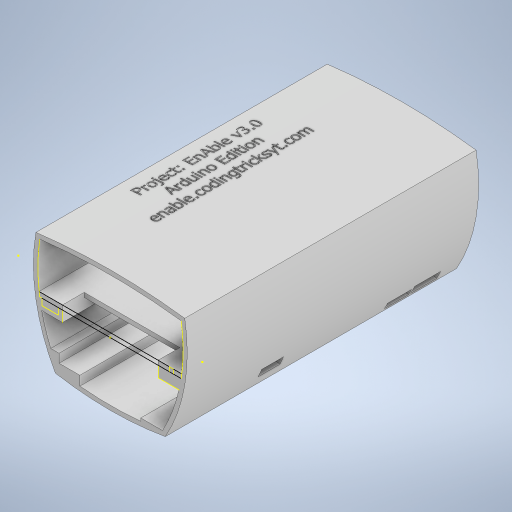
# Autodesk Inventor part: testingagain
Saved by Autodesk Inventor 2024 (Build 280153000, 153)
## iProperties
Created: 2022-11-19
Part Number: testingagain
Material: Generic
Document SubType Name: Modeling
Designer: jeron
Density: 1 g/cm^3
Appearance: Default
Author: jeron
Autodesk Inventor part; units mm, degrees
(part 1 of 2)
sketch "Sketch1" plane through (0, 0, 0) normal (0, 0, 1) x (1, 0, 0)
  line L0 (-32.5, 23) -> (32.5, 23)
  line L1 (32.5, 23) -> (32.5, 0)
  line L2 (-32.5, 0) -> (-32.5, 23)
  line L3 (-24, -18) -> (-24, 0)
  line L4 (24, -25) -> (24, -5)
  line L5 (0, -25) -> (24, -25)
  line L6 (0, -25) -> (-14, -25)
  line L7 (0, 23) -> (0, 25)
  line L8 (0, -25) -> (0, -27)
  arc A0 (-32.5, 23) -> (-24, -25) centre (42.3382, 11.5) ccw
  line L9 (-32.5, 0) -> (-31.5587, 0)
  line L10 (-24, 0) -> (-24, -5)
  line L11 (32.5, 0) -> (24, 0)
  line L12 (24, 0) -> (24, -5)
  line L13 (24, -5) -> (31.5587, -5)
  line L14 (24, -25) -> (15.6259, -25)
  line L15 (24, -25) -> (14, -25)
  line L16 (14, -25) -> (14, -26.3226)
  line L17 (-14, -25) -> (-14, -26.3226)
  arc A1 (32.5, 23) -> (-32.5, 23) centre (0, -240.0625) ccw
  arc A2 (24, -25) -> (32.5, 23) centre (-42.3382, 11.5) ccw
  arc A3 (-24, -25) -> (24, -25) centre (0, 118) ccw
  arc A4 (-34.2324, 24.7969) -> (-25.28, -26.8099) centre (42.3382, 11.5) ccw
  arc A5 (-25.28, -26.8099) -> (25.28, -26.8099) centre (0, 118) ccw
  arc A6 (25.28, -26.8099) -> (34.2324, 24.7969) centre (-42.3382, 11.5) ccw
  arc A7 (34.2324, 24.7969) -> (-34.2324, 24.7969) centre (0, -240.0625) ccw
  line L18 (-14, -25) -> (-14, -22)
  line L19 (-14, -22) -> (-25.5644, -22)
  line L20 (-24, -5) -> (-22, -5)
  line L21 (-22, -5) -> (-22, 0)
  line L22 (-31.5587, -5) -> (-31.5587, 0)
  line L23 (-32.5, 0) -> (-31.5587, 0)
  line L24 (-24, 0) -> (32.5, 0)
  line L25 (24, -5) -> (22, -5)
  line L26 (22, -5) -> (22, 0)
  line L27 (24, 0) -> (27, 0)
  line L28 (27, 0) -> (27, 2)
  line L29 (27, 2) -> (29, 2)
  line L30 (29, 2) -> (29, 0)
  line L31 (27, 0) -> (29, 0)
  line L32 (-25.5644, -22) -> (-23.5644, -22)
  line L33 (-23.5644, -22) -> (-23.5644, -18)
  line L34 (-23.5644, -18) -> (-27.3953, -18)
  line L35 (-24, -5) -> (-24, -3)
  line L36 (-24, -3) -> (-31.977, -3)
  line L37 (-24, -5) -> (-31.5587, -5)
  line L38 (0, 0) -> (0, -1.7837)
  point P0 (0, -28)
  point P1 (0, 26)
  point P2 (27, 0)
  point P3 (29, 0)
  point P4 (-31.5587, -3)
  point P5 (0, -29)
  point P6 (0, -27)
  point P7 (0, 27)
  point P8 (0, 25)
  dimension "d19" = 65
  dimension "d20" = 23
  dimension "d30" = 65
  dimension "d39" = 48
  dimension "d40" = 25
  dimension "d41" = 8.5
  dimension "d42" = 8.5
  dimension "d43" = 2
  dimension "d44" = 2
  dimension "d45" = 54
  dimension "d46" = 5
  dimension "d47" = 5
  dimension "d48" = 10
  dimension "d49" = 10
  dimension "d54" = 3
  dimension "d55" = 2
  dimension "d56" = 2
  dimension "d68" = 3
  dimension "d69" = 2
  dimension "d70" = 2
  dimension "d84" = 2
  dimension "d85" = 4
  dimension "d88" = 2
  dimension "d123" = 23
  dimension "d124" = 25
  dimension "d125" = 32.5
  dimension "d126" = 2
  dimension "d127" = 2
  constraints: 78 end point, 28 point on circle, 14 perpendicular, 12 point on line, 8 centre point, 7 horizontal, 4 collinear, 4 vertical, 1 midpoint, 1 parallel, 3 other
  measures "d19" distance of L0.start L0.end
  measures "d20" distance of L0.end L1.end
  measures "d30" distance of L1.end L2.start
  measures "d39" distance of L11.end L3.end
  measures "d40" distance of L4.start L11.end
  measures "d41" distance of L11.end L1.end
  measures "d42" distance of L2.start L3.end
  measures "d43" distance of L7.start L7.end
  measures "d44" distance of L5.start L8.end
  measures "d45" distance of point (0, -28) point (0, 26)
  measures "d46" distance of L3.end L10.end
  measures "d47" distance of L4.end L11.end
  measures "d48" distance of L14.start L15.end
  measures "d49" distance of L6.end A0.end
  measures "d54" distance of L6.end L18.end
  measures "d55" distance of L10.end L20.end
  measures "d56" distance of L4.end L25.end
  measures "d68" distance of L11.end L27.end
  measures "d69" distance of L27.end L28.end
  measures "d70" distance of L28.end L29.end
  measures "d84" distance of L19.end L32.end
  measures "d85" distance of L32.end L33.end
  measures "d88" distance of L10.end L35.end
  measures "d123" distance between parallel lines of L0 L24
  measures "d124" distance between parallel lines of L6 L24
  measures "d125" distance of L38.start L1.end
  measures "d126" distance of point (0, -29) point (0, -27)
  measures "d127" distance of point (0, 27) point (0, 25)
extrude "Extrusion3" add sketch "Sketch1" along normal blind 100 contours L9 L22 L36 A0 | L36 L22 A0 | A2 L13 L12 L11 | L3 L24 L21 L20 | L25 L26 L24 L12 | A3 L16 L5 | L19 L18 L17 A3 A0 | A7 A6 A5 A4
extrude "Extrusion4" add sketch "Sketch1" against normal blind 2 contours A1 L7 L0 | L0 L1 L11 L30 L29 L28 L24 L3 L36 L22 L9 L2 | L2 A0 | L7 A1 L0 | L9 L22 L36 A0 | A2 L1 | L36 L22 A0 | A2 L13 L12 L11 | L37 L3 L34 A0 | L22 L36 L3 L37 | L11 L28 L29 L30 | A2 L4 L13 | L34 L33 L19 A0 | L20 L21 L24 L26 L25 L4 L5 L6 L18 L19 L33 L34 L3 | L3 L24 L21 L20 | L25 L26 L24 L12 | A3 L16 L5 | L19 L18 L17 A3 A0 | A3 L8 L5 L16 | A3 L17 L6 L8 | A7 A6 A5 A4
ref_plane "Work Plane2" through (0, 27, 100) normal (0, 1, 0) x (-1, 0, 0)
sketch "Sketch3" plane through (0, 0, 0) normal (0, 0, 1) x (1, 0, 0)
  point P0 (0, 0)
ref_plane "Work Plane4" through (34.2348, -1.7834, -2) normal (0.9852847, -0.1709212, 0) x (0.1709212, 0.9852847, 0)
sketch "Sketch5" plane through (34.2348, -1.7834, -2) normal (0.9852847, -0.1709212, 0) x (0.1709212, 0.9852847, 0)
  line L0 (-24.6243, 2) -> (-24.6243, 102) projected
  line L1 (-24.6243, 2) -> (-24.6243, 10)
  line L2 (-24.6243, 10) -> (-20.6243, 10)
  line L3 (-20.6243, 10) -> (-20.6243, 22)
  line L4 (-20.6243, 22) -> (-24.6243, 22)
  line L5 (-24.6243, 22) -> (-24.6243, 23)
  line L6 (-24.6243, 23) -> (-21.6243, 23)
  line L7 (-21.6243, 23) -> (-21.6243, 34)
  line L8 (-21.6243, 34) -> (-24.6243, 34)
  line L9 (-24.6243, 2) -> (-24.6243, 84)
  line L10 (-24.6243, 84) -> (-16.6243, 84)
  line L11 (-16.6243, 84) -> (-16.6243, 94)
  line L12 (-16.6243, 94) -> (-24.6243, 94)
  line L13 (-24.6243, 84) -> (-20.6243, 84)
  line L14 (-20.6243, 84) -> (-20.6243, 94)
  point P0 (-4.0943, 2)
  dimension "d76" = 8
  dimension "d77" = 4
  dimension "d78" = 12
  dimension "d79" = 1
  dimension "d80" = 3
  dimension "d81" = 11
  dimension "d91" = 82
  dimension "d92" = 8
  dimension "d93" = 10
  dimension "d94" = 4
  constraints: 28 end point, 8 perpendicular, 6 point on line, 2 midpoint, 1 vertical
  measures "d76" distance of L0.start L1.end
  measures "d77" distance of L1.end L2.end
  measures "d78" distance of L2.end L3.end
  measures "d79" distance of L4.end L5.end
  measures "d80" distance of L5.end L6.end
  measures "d81" distance of L6.end L7.end
  measures "d91" distance of L0.start L9.end
  measures "d92" distance of L9.end L10.end
  measures "d93" distance of L10.end L11.end
  measures "d94" distance of L9.end L13.end
extrude "Extrusion7" cut sketch "Sketch5" against normal blind 10 contours L0 L4 L3 L2 | L0 L8 L7 L6 | L14 L12 L11 L10
extrude "Extrusion8" add sketch "Sketch1" along normal up to surface (100 mm away) contours L11 L28 L29 L30 | L34 L33 L19 A0
extrude "Extrusion9" add sketch "Sketch1" along normal up to surface (100 mm away) contours L22 L36 L3 L37
ref_plane "Work Plane5" through (-34.2348, -1.7834, 100) normal (-0.9852847, -0.1709212, 0) x (0.1709212, -0.9852847, 0)
sketch "Sketch6" plane through (-34.2348, -1.7834, 100) normal (-0.9852847, -0.1709212, 0) x (0.1709212, -0.9852847, 0)
  line L0 (17.147, 0) -> (17.147, -100) projected
  line L1 (17.147, -100) -> (17.147, -18)
  line L2 (17.147, -18) -> (13.147, -18)
  line L3 (13.147, -18) -> (13.147, -8)
  line L4 (13.147, -8) -> (17.147, -8)
  point P0 (4.0943, -100)
  dimension "d95" = 82
  dimension "d96" = 4
  dimension "d97" = 10
  constraints: 8 end point, 3 perpendicular, 2 point on line
  measures "d95" distance of L0.end L1.end
  measures "d96" distance of L1.end L2.end
  measures "d97" distance of L2.end L3.end
extrude "Extrusion10" cut sketch "Sketch6" against normal blind 10
ref_plane "Work Plane6" through (34.2324, 24.7969, 100) normal (0, 0, 1) x (1, 0, 0)
sketch "Sketch7" plane through (34.2324, 24.7969, 100) normal (0, 0, 1) x (1, 0, 0)
  arc A0 (0, 0) -> (-68.4649, 0) centre (-34.2324, -264.8594) ccw projected
  arc A1 (-68.4649, 0) -> (-59.5124, -51.6069) centre (8.1058, -13.2969) ccw projected
  arc A2 (-66.7324, -1.7969) -> (-66.7324, -24.7969) centre (8.1058, -13.2969) ccw projected
  arc A3 (-1.7324, -1.7969) -> (-66.7324, -1.7969) centre (-34.2324, -264.8594) ccw projected
  arc A4 (-8.9524, -51.6069) -> (0, 0) centre (-76.5707, -13.2969) ccw projected
  arc A5 (-1.7324, -24.7969) -> (-1.7324, -1.7969) centre (-76.5707, -13.2969) ccw projected
  line L0 (-1.7324, -24.7969) -> (-5.2324, -24.7969) projected
  line L1 (-5.2324, -22.7969) -> (-5.2324, -24.7969) projected
  line L2 (-7.2324, -22.7969) -> (-5.2324, -22.7969) projected
  line L3 (-7.2324, -24.7969) -> (-7.2324, -22.7969) projected
  line L4 (-7.2324, -24.7969) -> (-12.2324, -24.7969) projected
  line L5 (-12.2324, -24.7969) -> (-12.2324, -29.7969) projected
  line L6 (-12.2324, -29.7969) -> (-2.6737, -29.7969) projected
  arc A6 (-10.2324, -49.7969) -> (-2.6737, -29.7969) centre (-76.5707, -13.2969) ccw projected
  line L7 (-65.7912, -24.7969) -> (-66.7324, -24.7969) projected
  line L8 (-65.7912, -27.7969) -> (-65.7912, -24.7969) projected
  line L9 (-65.7912, -27.7969) -> (-58.2324, -27.7969) projected
  line L10 (-58.2324, -24.7969) -> (-58.2324, -27.7969) projected
  line L11 (-56.2324, -24.7969) -> (-58.2324, -24.7969) projected
  line L12 (-56.2324, -29.7969) -> (-56.2324, -24.7969) projected
  line L13 (-56.2324, -29.7969) -> (-65.7912, -29.7969) projected
  arc A7 (-65.7912, -29.7969) -> (-61.6277, -42.7969) centre (8.1058, -13.2969) ccw projected
  line L14 (-61.6277, -42.7969) -> (-57.7968, -42.7969) projected
  line L15 (-57.7968, -42.7969) -> (-57.7968, -46.7969) projected
  line L16 (-48.2324, -46.7969) -> (-57.7968, -46.7969) projected
  line L17 (-48.2324, -51.1195) -> (-48.2324, -46.7969) projected
  arc A8 (-48.2324, -51.1195) -> (-20.2324, -51.1195) centre (-34.2324, 93.2031) ccw projected
  line L18 (-20.2324, -49.7969) -> (-20.2324, -51.1195) projected
  line L19 (-10.2324, -49.7969) -> (-20.2324, -49.7969) projected
  arc A9 (-59.5124, -51.6069) -> (-8.9524, -51.6069) centre (-34.2324, 93.2031) ccw projected
  point P0 (-34.2324, -24.7969)
extrude "Extrusion11" add sketch "Sketch7" along normal blind 32
sketch "Sketch8" plane through (0, 0, -2) normal (0, 0, -1) x (-1, 0, 0)
  circle A0 centre (0, 0) radius 16
  arc A1 (30.7676, 23.2082) -> (-24.2324, 23.89) centre (0, -240.0625) ccw projected
  line L0 (30.7676, 23.2082) -> (7.9501, 23.2082)
  line L1 (7.9501, 23.2082) -> (7.9501, 13.8851)
  line L2 (15.0321, 5.4805) -> (30.7676, 5.4805)
  line L3 (30.7676, 5.4805) -> (30.7676, 23.2082)
  circle A2 centre (0, 10) radius 1.5
  circle A3 centre (0, -10) radius 1.5
  dimension "d102" = 32
  dimension "d104" = 3
  dimension "d106" = 3
  dimension "d121" = 10
  dimension "d122" = 10
  dimension "d128" = 7.9501
  dimension "d129" = 13.8851
  dimension "d130" = 22.8175
  dimension "d131" = 17.7278
  constraints: 8 end point, 3 centre point, 2 horizontal, 2 perpendicular, 2 point on circle, 1 coincident
  measures "d102" diameter of A0
  measures "d104" diameter of A2
  measures "d106" diameter of A3
  measures "d121" distance of point (0, 0) A2.centre
  measures "d122" distance of point (0, 0) A3.centre
  measures "d128" horizontal distance of point (0, 0) L1.end
  measures "d129" vertical distance of point (0, 0) L1.end
  measures "d130" distance of L0.end L0.start
  measures "d131" distance of L2.end L0.start
extrude "Extrusion12" cut sketch "Sketch8" against normal up to surface (2 mm away) contours A0 L1 L0 L3 L2 | A2 | A3
sketch "Sketch9" plane through (34.2324, 24.7969, 132) normal (0, 0, 1) x (1, 0, 0)
  point P0 (-34.2324, -24.7969)
sketch "Sketch11" plane through (34.2324, 24.7969, 132) normal (0, 0, 1) x (1, 0, 0)
  line L0 (-65.7912, -24.7969) -> (-66.7324, -24.7969) projected
  line L1 (-7.2324, -24.7969) -> (-12.2324, -24.7969) projected
  line L2 (-65.7912, -24.7969) -> (-7.2324, -24.7969)
  arc A0 (-1.7324, -24.7969) -> (-1.7324, -1.7969) centre (-76.5707, -13.2969) ccw projected
  line L3 (-7.2324, -24.7969) -> (-1.7324, -24.7969)
  line L4 (-56.2324, -29.7969) -> (-56.2324, -24.7969) projected
  line L5 (-12.2324, -29.7969) -> (-2.6737, -29.7969) projected
  line L6 (-58.2324, -27.7969) -> (-65.7912, -27.7969) projected
  line L7 (-58.2324, -24.7969) -> (-58.2324, -27.7969) projected
  line L8 (-65.7912, -27.7969) -> (-65.7912, -24.7969) projected
  line L9 (-7.2324, -22.7969) -> (-7.2324, -24.7969) projected
  line L10 (-5.2324, -22.7969) -> (-7.2324, -22.7969) projected
  line L11 (-5.2324, -24.7969) -> (-5.2324, -22.7969) projected
  line L12 (-12.2324, -24.7969) -> (-12.2324, -29.7969) projected
  line L13 (-5.2324, -22.7969) -> (-1.4524, -22.7969)
  line L14 (-7.2324, -22.7969) -> (-67.0125, -22.7969)
  arc A1 (-66.7324, -1.7969) -> (-66.7324, -24.7969) centre (8.1058, -13.2969) ccw projected
  point P0 (-34.2324, -24.7969)
  constraints: 8 end point, 2 point on circle, 1 collinear, 1 horizontal, 1 parallel, 1 point on line
extrude "Extrusion15" add sketch "Sketch11" against normal up to surface (132 mm away) contours L2 L7 L6 L8
ref_plane "Work Plane7" through (0, 27, -2) normal (0, 1, 0) x (-1, 0, 0)
sketch "Sketch14" plane through (0, 27, -2) normal (0, 1, 0) x (-1, 0, 0)
  line L0 (28.7956, 103.5089) -> (28.7956, 32.4114) construction
  line L1 (28.7956, 32.4114) -> (-135.0036, 32.4114) construction
  line L2 (-135.0036, 32.4114) -> (-135.0036, 103.5089) construction
  line L3 (-135.0036, 103.5089) -> (28.7956, 103.5089) construction
  spline S0 degree 2 poles (27.1788, 93.3054) (26.8759, 93.3054) (26.3306, 93.5212) (26.1413, 93.7143) knots 0 0 0 1 2 2 2
  spline S1 degree 2 poles (26.1413, 93.7143) (25.9027, 93.9566) (25.6566, 94.6117) (25.6566, 95.1115) knots 0 0 0 1 2 2 2
  line L4 (25.6566, 95.1115) -> (25.6566, 95.6379)
  line L5 (25.6566, 95.6379) -> (23.9148, 95.6379)
  line L6 (23.9148, 95.6379) -> (23.9148, 96.2588)
  line L7 (23.9148, 96.2588) -> (28.5874, 96.2588)
  line L8 (28.5874, 96.2588) -> (28.5874, 95.085)
  spline S2 degree 2 poles (28.5874, 95.085) (28.5874, 94.6685) (28.4511, 94.0854) (28.2958, 93.862) knots 0 0 0 1 2 2 2
  spline S3 degree 2 poles (28.2958, 93.862) (28.1178, 93.6007) (27.5688, 93.3054) (27.1788, 93.3054) knots 0 0 0 1 2 2 2
  spline S4 degree 2 poles (27.1598, 93.9528) (27.4022, 93.9528) (27.7581, 94.1195) (27.8717, 94.2898) knots 0 0 0 1 2 2 2
  spline S5 degree 2 poles (27.8717, 94.2898) (27.9702, 94.4375) (28.0497, 94.8313) (28.0497, 95.1229) knots 0 0 0 1 2 2 2
  line L9 (28.0497, 95.1229) -> (28.0497, 95.6379)
  line L10 (28.0497, 95.6379) -> (26.1867, 95.6379)
  line L11 (26.1867, 95.6379) -> (26.1867, 95.2138)
  spline S6 degree 2 poles (26.1867, 95.2138) (26.1867, 94.8351) (26.3079, 94.3694) (26.4669, 94.2179) knots 0 0 0 1 2 2 2
  spline S7 degree 2 poles (26.4669, 94.2179) (26.607, 94.0778) (26.9364, 93.9528) (27.1598, 93.9528) knots 0 0 0 1 2 2 2
  line L12 (26.7888, 90.9009) -> (26.7888, 90.9312)
  spline S8 degree 2 poles (26.7888, 90.9312) (26.8077, 90.9994) (26.8153, 91.147) (26.8153, 91.2493) knots 0 0 0 1 2 2 2
  spline S9 degree 2 poles (26.8153, 91.2493) (26.8153, 91.4878) (26.607, 91.9573) (26.4025, 92.1694) knots 0 0 0 1 2 2 2
  line L13 (26.4025, 92.1694) -> (23.9148, 92.1694)
  line L14 (23.9148, 92.1694) -> (23.9148, 92.7601)
  line L15 (23.9148, 92.7601) -> (27.4211, 92.7601)
  line L16 (27.4211, 92.7601) -> (27.4211, 92.1694)
  line L17 (27.4211, 92.1694) -> (26.8986, 92.1694)
  spline S10 degree 2 poles (26.8986, 92.1694) (27.1863, 91.8475) (27.4211, 91.3666) (27.4211, 91.1395) knots 0 0 0 1 2 2 2
  spline S11 degree 2 poles (27.4211, 91.1395) (27.4211, 91.0486) (27.4135, 90.9577) (27.4022, 90.9009) knots 0 0 0 1 2 2 2
  line L18 (27.4022, 90.9009) -> (26.7888, 90.9009)
  spline S12 degree 2 poles (25.6679, 87.5612) (24.7819, 87.5612) (23.8163, 88.4131) (23.8163, 89.125) knots 0 0 0 1 2 2 2
  spline S13 degree 2 poles (23.8163, 89.125) (23.8163, 89.8558) (24.8122, 90.6926) (25.6679, 90.6926) knots 0 0 0 1 2 2 2
  spline S14 degree 2 poles (25.6679, 90.6926) (26.5464, 90.6926) (27.5196, 89.8293) (27.5196, 89.125) knots 0 0 0 1 2 2 2
  spline S15 degree 2 poles (27.5196, 89.125) (27.5196, 88.4131) (26.5502, 87.5612) (25.6679, 87.5612) knots 0 0 0 1 2 2 2
  spline S16 degree 2 poles (25.6679, 88.1708) (26.3495, 88.1708) (27.0122, 88.6668) (27.0122, 89.125) knots 0 0 0 1 2 2 2
  spline S17 degree 2 poles (27.0122, 89.125) (27.0122, 89.5832) (26.3495, 90.083) (25.6679, 90.083) knots 0 0 0 1 2 2 2
  spline S18 degree 2 poles (25.6679, 90.083) (25.0053, 90.083) (24.3237, 89.5832) (24.3237, 89.125) knots 0 0 0 1 2 2 2
  spline S19 degree 2 poles (24.3237, 89.125) (24.3237, 88.6706) (24.9939, 88.1708) (25.6679, 88.1708) knots 0 0 0 1 2 2 2
  spline S20 degree 2 poles (23.8163, 86.0011) (23.2181, 86.0011) (22.5895, 86.6448) (22.5895, 87.209) knots 0 0 0 1 2 2 2
  spline S21 degree 2 poles (22.5895, 87.209) (22.5895, 87.3075) (22.6084, 87.5498) (22.6274, 87.6672) knots 0 0 0 1 2 2 2
  line L19 (22.6274, 87.6672) -> (23.1575, 87.6672)
  line L20 (23.1575, 87.6672) -> (23.1575, 87.6331)
  spline S22 degree 2 poles (23.1575, 87.6331) (23.1423, 87.565) (23.112, 87.3984) (23.112, 87.3226) knots 0 0 0 1 2 2 2
  spline S23 degree 2 poles (23.112, 87.3226) (23.112, 87.0879) (23.2294, 86.7812) (23.3544, 86.7092) knots 0 0 0 1 2 2 2
  spline S24 degree 2 poles (23.3544, 86.7092) (23.468, 86.6373) (23.8125, 86.5918) (24.0587, 86.5918) knots 0 0 0 1 2 2 2
  line L21 (24.0587, 86.5918) -> (26.9327, 86.5918)
  line L22 (26.9327, 86.5918) -> (26.9327, 87.2242)
  line L23 (26.9327, 87.2242) -> (27.4211, 87.2242)
  line L24 (27.4211, 87.2242) -> (27.4211, 86.0011)
  line L25 (27.4211, 86.0011) -> (23.8163, 86.0011)
  line L26 (28.0042, 85.9973) -> (28.0042, 86.6676)
  line L27 (28.0042, 86.6676) -> (28.6177, 86.6676)
  line L28 (28.6177, 86.6676) -> (28.6177, 85.9973)
  line L29 (28.6177, 85.9973) -> (28.0042, 85.9973)
  spline S25 degree 2 poles (23.8353, 83.6232) (23.8353, 84.4638) (24.7781, 85.3877) (25.649, 85.3877) knots 0 0 0 1 2 2 2
  spline S26 degree 2 poles (25.649, 85.3877) (26.5048, 85.3877) (27.5196, 84.4903) (27.5196, 83.7671) knots 0 0 0 1 2 2 2
  spline S27 degree 2 poles (27.5196, 83.7671) (27.5196, 83.4414) (27.3302, 82.9378) (27.1296, 82.7523) knots 0 0 0 1 2 2 2
  spline S28 degree 2 poles (27.1296, 82.7523) (26.9289, 82.563) (26.3495, 82.3623) (25.9292, 82.3623) knots 0 0 0 1 2 2 2
  line L30 (25.9292, 82.3623) -> (25.6074, 82.3623)
  line L31 (25.6074, 82.3623) -> (25.6074, 84.7894)
  spline S29 degree 2 poles (25.6074, 84.7894) (24.9977, 84.7894) (24.3502, 84.176) (24.3502, 83.6308) knots 0 0 0 1 2 2 2
  spline S30 degree 2 poles (24.3502, 83.6308) (24.3502, 83.4376) (24.4373, 83.0628) (24.5055, 82.9113) knots 0 0 0 1 2 2 2
  spline S31 degree 2 poles (24.5055, 82.9113) (24.5812, 82.7523) (24.7137, 82.5327) (24.7743, 82.4607) knots 0 0 0 1 2 2 2
  line L32 (24.7743, 82.4607) -> (24.7743, 82.4266)
  line L33 (24.7743, 82.4266) -> (24.1306, 82.4266)
  spline S32 degree 2 poles (24.1306, 82.4266) (24.089, 82.5289) (23.9678, 82.8394) (23.9337, 82.9605) knots 0 0 0 1 2 2 2
  spline S33 degree 2 poles (23.9337, 82.9605) (23.8845, 83.1309) (23.8353, 83.4111) (23.8353, 83.6232) knots 0 0 0 1 2 2 2
  spline S34 degree 2 poles (26.058, 82.9378) (26.2965, 82.9454) (26.6449, 83.0438) (26.7623, 83.1385) knots 0 0 0 1 2 2 2
  spline S35 degree 2 poles (26.7623, 83.1385) (26.8948, 83.2407) (27.0349, 83.5626) (27.0349, 83.8011) knots 0 0 0 1 2 2 2
  spline S36 degree 2 poles (27.0349, 83.8011) (27.0349, 84.0359) (26.8948, 84.3653) (26.7585, 84.5017) knots 0 0 0 1 2 2 2
  spline S37 degree 2 poles (26.7585, 84.5017) (26.6184, 84.6342) (26.2814, 84.7705) (26.058, 84.7894) knots 0 0 0 1 2 2 2
  line L34 (26.058, 84.7894) -> (26.058, 82.9378)
  spline S38 degree 2 poles (23.8353, 80.3705) (23.8353, 80.7341) (24.0587, 81.3361) (24.2859, 81.5519) knots 0 0 0 1 2 2 2
  spline S39 degree 2 poles (24.2859, 81.5519) (24.5093, 81.7678) (25.1984, 82.0063) (25.6604, 82.0063) knots 0 0 0 1 2 2 2
  spline S40 degree 2 poles (25.6604, 82.0063) (26.1223, 82.0063) (26.7963, 81.7602) (27.0235, 81.5519) knots 0 0 0 1 2 2 2
  spline S41 degree 2 poles (27.0235, 81.5519) (27.2545, 81.3437) (27.5006, 80.7265) (27.5006, 80.3705) knots 0 0 0 1 2 2 2
  spline S42 degree 2 poles (27.5006, 80.3705) (27.5006, 80.0828) (27.3378, 79.5451) (27.2318, 79.3368) knots 0 0 0 1 2 2 2
  line L35 (27.2318, 79.3368) -> (26.5691, 79.3368)
  line L36 (26.5691, 79.3368) -> (26.5691, 79.3709)
  spline S43 degree 2 poles (26.5691, 79.3709) (26.6222, 79.4353) (26.7585, 79.6322) (26.8304, 79.7723) knots 0 0 0 1 2 2 2
  spline S44 degree 2 poles (26.8304, 79.7723) (26.891, 79.8972) (26.9857, 80.2304) (26.9857, 80.3819) knots 0 0 0 1 2 2 2
  spline S45 degree 2 poles (26.9857, 80.3819) (26.9857, 80.8401) (26.2927, 81.3967) (25.6604, 81.3967) knots 0 0 0 1 2 2 2
  spline S46 degree 2 poles (25.6604, 81.3967) (25.0432, 81.3967) (24.3502, 80.859) (24.3502, 80.3819) knots 0 0 0 1 2 2 2
  spline S47 degree 2 poles (24.3502, 80.3819) (24.3502, 80.0941) (24.5888, 79.5716) (24.7743, 79.3709) knots 0 0 0 1 2 2 2
  line L37 (24.7743, 79.3709) -> (24.7743, 79.3368)
  line L38 (24.7743, 79.3368) -> (24.1117, 79.3368)
  spline S48 degree 2 poles (24.1117, 79.3368) (24.07, 79.4239) (23.9526, 79.689) (23.9261, 79.795) knots 0 0 0 1 2 2 2
  spline S49 degree 2 poles (23.9261, 79.795) (23.8807, 79.9465) (23.8353, 80.185) (23.8353, 80.3705) knots 0 0 0 1 2 2 2
  spline S50 degree 2 poles (23.8466, 77.7389) (23.8466, 78.2198) (24.3957, 78.7613) (24.9902, 78.7613) knots 0 0 0 1 2 2 2
  line L39 (24.9902, 78.7613) -> (26.9327, 78.7613)
  line L40 (26.9327, 78.7613) -> (26.9327, 79.1589)
  line L41 (26.9327, 79.1589) -> (27.4211, 79.1589)
  line L42 (27.4211, 79.1589) -> (27.4211, 78.7613)
  line L43 (27.4211, 78.7613) -> (28.4283, 78.7613)
  line L44 (28.4283, 78.7613) -> (28.4283, 78.1706)
  line L45 (28.4283, 78.1706) -> (27.4211, 78.1706)
  line L46 (27.4211, 78.1706) -> (27.4211, 77.0838)
  line L47 (27.4211, 77.0838) -> (26.9327, 77.0838)
  line L48 (26.9327, 77.0838) -> (26.9327, 78.1706)
  line L49 (26.9327, 78.1706) -> (25.2628, 78.1706)
  spline S51 degree 2 poles (25.2628, 78.1706) (24.9977, 78.1706) (24.7062, 78.1516) (24.5812, 78.0873) knots 0 0 0 1 2 2 2
  spline S52 degree 2 poles (24.5812, 78.0873) (24.4714, 78.0343) (24.3616, 77.7957) (24.3616, 77.5912) knots 0 0 0 1 2 2 2
  spline S53 degree 2 poles (24.3616, 77.5912) (24.3616, 77.4473) (24.4487, 77.1785) (24.4752, 77.1179) knots 0 0 0 1 2 2 2
  line L50 (24.4752, 77.1179) -> (24.4752, 77.0838)
  line L51 (24.4752, 77.0838) -> (23.9451, 77.0838)
  spline S54 degree 2 poles (23.9451, 77.0838) (23.8996, 77.2504) (23.8466, 77.5912) (23.8466, 77.7389) knots 0 0 0 1 2 2 2
  line L52 (23.9148, 75.5654) -> (23.9148, 76.3152)
  line L53 (23.9148, 76.3152) -> (24.8084, 76.3152)
  line L54 (24.8084, 76.3152) -> (24.8084, 75.5654)
  line L55 (24.8084, 75.5654) -> (23.9148, 75.5654)
  line L56 (26.5275, 75.5654) -> (26.5275, 76.3152)
  line L57 (26.5275, 76.3152) -> (27.4211, 76.3152)
  line L58 (27.4211, 76.3152) -> (27.4211, 75.5654)
  line L59 (27.4211, 75.5654) -> (26.5275, 75.5654)
  line L60 (23.9148, 72.3242) -> (28.5874, 72.3242)
  line L61 (28.5874, 72.3242) -> (28.5874, 69.401)
  line L62 (28.5874, 69.401) -> (28.0345, 69.401)
  line L63 (28.0345, 69.401) -> (28.0345, 71.7032)
  line L64 (28.0345, 71.7032) -> (26.7547, 71.7032)
  line L65 (26.7547, 71.7032) -> (26.7547, 69.5562)
  line L66 (26.7547, 69.5562) -> (26.2019, 69.5562)
  line L67 (26.2019, 69.5562) -> (26.2019, 71.7032)
  line L68 (26.2019, 71.7032) -> (24.4676, 71.7032)
  line L69 (24.4676, 71.7032) -> (24.4676, 69.401)
  line L70 (24.4676, 69.401) -> (23.9148, 69.401)
  line L71 (23.9148, 69.401) -> (23.9148, 72.3242)
  line L72 (23.9148, 66.012) -> (23.9148, 66.6027)
  line L73 (23.9148, 66.6027) -> (25.9141, 66.6027)
  spline S55 degree 2 poles (25.9141, 66.6027) (26.1564, 66.6027) (26.5729, 66.6481) (26.6979, 66.7163) knots 0 0 0 1 2 2 2
  spline S56 degree 2 poles (26.6979, 66.7163) (26.8304, 66.7882) (26.9592, 67.0457) (26.9592, 67.2654) knots 0 0 0 1 2 2 2
  spline S57 degree 2 poles (26.9592, 67.2654) (26.9592, 67.485) (26.7244, 67.9507) (26.5351, 68.1741) knots 0 0 0 1 2 2 2
  line L74 (26.5351, 68.1741) -> (23.9148, 68.1741)
  line L75 (23.9148, 68.1741) -> (23.9148, 68.7648)
  line L76 (23.9148, 68.7648) -> (27.4211, 68.7648)
  line L77 (27.4211, 68.7648) -> (27.4211, 68.1741)
  line L78 (27.4211, 68.1741) -> (27.0311, 68.1741)
  spline S58 degree 2 poles (27.0311, 68.1741) (27.2697, 67.9091) (27.5196, 67.3979) (27.5196, 67.1101) knots 0 0 0 1 2 2 2
  spline S59 degree 2 poles (27.5196, 67.1101) (27.5196, 66.5951) (26.838, 66.012) (26.1905, 66.012) knots 0 0 0 1 2 2 2
  line L79 (26.1905, 66.012) -> (23.9148, 66.012)
  line L80 (23.9148, 65.6409) -> (28.5874, 64.0657)
  line L81 (28.5874, 64.0657) -> (28.5874, 63.3008)
  line L82 (28.5874, 63.3008) -> (23.9148, 61.7257)
  line L83 (23.9148, 61.7257) -> (23.9148, 62.3807)
  line L84 (23.9148, 62.3807) -> (25.2211, 62.8048)
  line L85 (25.2211, 62.8048) -> (25.2211, 64.5883)
  line L86 (25.2211, 64.5883) -> (23.9148, 65.0124)
  line L87 (23.9148, 65.0124) -> (23.9148, 65.6409)
  line L88 (25.7513, 62.9752) -> (27.9512, 63.6984)
  line L89 (27.9512, 63.6984) -> (25.7513, 64.4179)
  line L90 (25.7513, 64.4179) -> (25.7513, 62.9752)
  spline S60 degree 2 poles (25.7247, 58.3897) (24.8652, 58.3897) (23.8163, 59.2228) (23.8163, 59.8513) knots 0 0 0 1 2 2 2
  spline S61 degree 2 poles (23.8163, 59.8513) (23.8163, 60.1353) (23.9564, 60.5405) (24.0776, 60.7374) knots 0 0 0 1 2 2 2
  line L91 (24.0776, 60.7374) -> (23.9148, 60.7752)
  line L92 (23.9148, 60.7752) -> (23.9148, 61.3281)
  line L93 (23.9148, 61.3281) -> (28.7956, 61.3281)
  line L94 (28.7956, 61.3281) -> (28.7956, 60.7374)
  line L95 (28.7956, 60.7374) -> (27.0538, 60.7374)
  spline S62 degree 2 poles (27.0538, 60.7374) (27.2545, 60.514) (27.5196, 59.9952) (27.5196, 59.6658) knots 0 0 0 1 2 2 2
  spline S63 degree 2 poles (27.5196, 59.6658) (27.5196, 59.0713) (26.5691, 58.3897) (25.7247, 58.3897) knots 0 0 0 1 2 2 2
  spline S64 degree 2 poles (25.6793, 58.9993) (26.3079, 58.9993) (26.9592, 59.3818) (26.9592, 59.8059) knots 0 0 0 1 2 2 2
  spline S65 degree 2 poles (26.9592, 59.8059) (26.9592, 60.0444) (26.732, 60.5367) (26.5578, 60.7374) knots 0 0 0 1 2 2 2
  line L96 (26.5578, 60.7374) -> (24.5471, 60.7374)
  spline S66 degree 2 poles (24.5471, 60.7374) (24.4373, 60.514) (24.3464, 60.1694) (24.3464, 59.9649) knots 0 0 0 1 2 2 2
  spline S67 degree 2 poles (24.3464, 59.9649) (24.3464, 59.5143) (24.9864, 58.9993) (25.6793, 58.9993) knots 0 0 0 1 2 2 2
  line L97 (23.9148, 57.1742) -> (23.9148, 57.7649)
  line L98 (23.9148, 57.7649) -> (28.7956, 57.7649)
  line L99 (28.7956, 57.7649) -> (28.7956, 57.1742)
  line L100 (28.7956, 57.1742) -> (23.9148, 57.1742)
  spline S68 degree 2 poles (23.8353, 54.7849) (23.8353, 55.6255) (24.7781, 56.5495) (25.649, 56.5495) knots 0 0 0 1 2 2 2
  spline S69 degree 2 poles (25.649, 56.5495) (26.5048, 56.5495) (27.5196, 55.652) (27.5196, 54.9288) knots 0 0 0 1 2 2 2
  spline S70 degree 2 poles (27.5196, 54.9288) (27.5196, 54.6032) (27.3302, 54.0996) (27.1296, 53.914) knots 0 0 0 1 2 2 2
  spline S71 degree 2 poles (27.1296, 53.914) (26.9289, 53.7247) (26.3495, 53.524) (25.9292, 53.524) knots 0 0 0 1 2 2 2
  line L101 (25.9292, 53.524) -> (25.6074, 53.524)
  line L102 (25.6074, 53.524) -> (25.6074, 55.9512)
  spline S72 degree 2 poles (25.6074, 55.9512) (24.9977, 55.9512) (24.3502, 55.3378) (24.3502, 54.7925) knots 0 0 0 1 2 2 2
  spline S73 degree 2 poles (24.3502, 54.7925) (24.3502, 54.5994) (24.4373, 54.2245) (24.5055, 54.0731) knots 0 0 0 1 2 2 2
  spline S74 degree 2 poles (24.5055, 54.0731) (24.5812, 53.914) (24.7137, 53.6944) (24.7743, 53.6225) knots 0 0 0 1 2 2 2
  line L103 (24.7743, 53.6225) -> (24.7743, 53.5884)
  line L104 (24.7743, 53.5884) -> (24.1306, 53.5884)
  spline S75 degree 2 poles (24.1306, 53.5884) (24.089, 53.6906) (23.9678, 54.0011) (23.9337, 54.1223) knots 0 0 0 1 2 2 2
  spline S76 degree 2 poles (23.9337, 54.1223) (23.8845, 54.2927) (23.8353, 54.5729) (23.8353, 54.7849) knots 0 0 0 1 2 2 2
  spline S77 degree 2 poles (26.058, 54.0996) (26.2965, 54.1071) (26.6449, 54.2056) (26.7623, 54.3003) knots 0 0 0 1 2 2 2
  spline S78 degree 2 poles (26.7623, 54.3003) (26.8948, 54.4025) (27.0349, 54.7243) (27.0349, 54.9629) knots 0 0 0 1 2 2 2
  spline S79 degree 2 poles (27.0349, 54.9629) (27.0349, 55.1977) (26.8948, 55.5271) (26.7585, 55.6634) knots 0 0 0 1 2 2 2
  spline S80 degree 2 poles (26.7585, 55.6634) (26.6184, 55.7959) (26.2814, 55.9323) (26.058, 55.9512) knots 0 0 0 1 2 2 2
  line L105 (26.058, 55.9512) -> (26.058, 54.0996)
  line L106 (27.4211, 48.1661) -> (23.9148, 49.4876)
  line L107 (23.9148, 49.4876) -> (23.9148, 50.0177)
  line L108 (23.9148, 50.0177) -> (27.4211, 51.3278)
  line L109 (27.4211, 51.3278) -> (27.4211, 50.6879)
  line L110 (27.4211, 50.6879) -> (24.7213, 49.7299)
  line L111 (24.7213, 49.7299) -> (27.4211, 48.7795)
  line L112 (27.4211, 48.7795) -> (27.4211, 48.1661)
  spline S81 degree 2 poles (28.1443, 46.5454) (28.1443, 46.7158) (28.061, 47.0528) (27.9967, 47.2156) knots 0 0 0 1 2 2 2
  spline S82 degree 2 poles (27.9967, 47.2156) (27.9323, 47.3671) (27.796, 47.5905) (27.7354, 47.6776) knots 0 0 0 1 2 2 2
  line L113 (27.7354, 47.6776) -> (27.7354, 47.7155)
  line L114 (27.7354, 47.7155) -> (28.398, 47.7155)
  spline S83 degree 2 poles (28.398, 47.7155) (28.5079, 47.511) (28.6858, 46.8105) (28.6858, 46.4962) knots 0 0 0 1 2 2 2
  spline S84 degree 2 poles (28.6858, 46.4962) (28.6858, 46.1781) (28.5571, 45.7048) (28.4208, 45.5117) knots 0 0 0 1 2 2 2
  spline S85 degree 2 poles (28.4208, 45.5117) (28.2731, 45.3072) (27.8452, 45.0952) (27.5574, 45.0952) knots 0 0 0 1 2 2 2
  spline S86 degree 2 poles (27.5574, 45.0952) (27.1712, 45.0952) (26.5881, 45.6026) (26.5123, 45.9585) knots 0 0 0 1 2 2 2
  line L115 (26.5123, 45.9585) -> (26.4669, 45.9585)
  spline S87 degree 2 poles (26.4669, 45.9585) (26.4366, 45.8108) (26.3003, 45.4738) (26.164, 45.33) knots 0 0 0 1 2 2 2
  spline S88 degree 2 poles (26.164, 45.33) (26.0315, 45.1861) (25.6074, 45.0043) (25.3007, 45.0043) knots 0 0 0 1 2 2 2
  spline S89 degree 2 poles (25.3007, 45.0043) (24.9864, 45.0043) (24.4525, 45.2201) (24.248, 45.417) knots 0 0 0 1 2 2 2
  spline S90 degree 2 poles (24.248, 45.417) (24.036, 45.6215) (23.8163, 46.2009) (23.8163, 46.5682) knots 0 0 0 1 2 2 2
  spline S91 degree 2 poles (23.8163, 46.5682) (23.8163, 46.9203) (23.9867, 47.6094) (24.1041, 47.8442) knots 0 0 0 1 2 2 2
  line L116 (24.1041, 47.8442) -> (24.7668, 47.8442)
  line L117 (24.7668, 47.8442) -> (24.7668, 47.7988)
  spline S92 degree 2 poles (24.7668, 47.7988) (24.6229, 47.6019) (24.3578, 46.9354) (24.3578, 46.606) knots 0 0 0 1 2 2 2
  spline S93 degree 2 poles (24.3578, 46.606) (24.3578, 46.4129) (24.479, 46.0267) (24.6191, 45.8979) knots 0 0 0 1 2 2 2
  spline S94 degree 2 poles (24.6191, 45.8979) (24.7592, 45.773) (25.0924, 45.6405) (25.3461, 45.6405) knots 0 0 0 1 2 2 2
  spline S95 degree 2 poles (25.3461, 45.6405) (25.5998, 45.6405) (25.9292, 45.7881) (26.0239, 45.9207) knots 0 0 0 1 2 2 2
  spline S96 degree 2 poles (26.0239, 45.9207) (26.1185, 46.0532) (26.1905, 46.4129) (26.1905, 46.6249) knots 0 0 0 1 2 2 2
  line L118 (26.1905, 46.6249) -> (26.1905, 46.89)
  line L119 (26.1905, 46.89) -> (26.7092, 46.89)
  line L120 (26.7092, 46.89) -> (26.7092, 46.6817)
  spline S97 degree 2 poles (26.7092, 46.6817) (26.7092, 46.2614) (27.1106, 45.7313) (27.4931, 45.7313) knots 0 0 0 1 2 2 2
  spline S98 degree 2 poles (27.4931, 45.7313) (27.671, 45.7313) (27.9247, 45.8676) (28.0005, 45.9775) knots 0 0 0 1 2 2 2
  spline S99 degree 2 poles (28.0005, 45.9775) (28.08, 46.0948) (28.1443, 46.3826) (28.1443, 46.5454) knots 0 0 0 1 2 2 2
  line L121 (23.9148, 43.2966) -> (23.9148, 44.0463)
  line L122 (23.9148, 44.0463) -> (24.8084, 44.0463)
  line L123 (24.8084, 44.0463) -> (24.8084, 43.2966)
  line L124 (24.8084, 43.2966) -> (23.9148, 43.2966)
  spline S100 degree 2 poles (26.2511, 39.4457) (24.9939, 39.4457) (23.8163, 40.1765) (23.8163, 40.9376) knots 0 0 0 1 2 2 2
  spline S101 degree 2 poles (23.8163, 40.9376) (23.8163, 41.71) (25.0167, 42.4333) (26.2473, 42.4333) knots 0 0 0 1 2 2 2
  spline S102 degree 2 poles (26.2473, 42.4333) (27.512, 42.4333) (28.682, 41.7025) (28.682, 40.9376) knots 0 0 0 1 2 2 2
  spline S103 degree 2 poles (28.682, 40.9376) (28.682, 40.1689) (27.4703, 39.4457) (26.2511, 39.4457) knots 0 0 0 1 2 2 2
  spline S104 degree 2 poles (24.8273, 40.2484) (25.0583, 40.1575) (25.7702, 40.0818) (26.2511, 40.0818) knots 0 0 0 1 2 2 2
  spline S105 degree 2 poles (26.2511, 40.0818) (26.732, 40.0818) (27.44, 40.1575) (27.6786, 40.2522) knots 0 0 0 1 2 2 2
  spline S106 degree 2 poles (27.6786, 40.2522) (27.9172, 40.3469) (28.1633, 40.6763) (28.1633, 40.9376) knots 0 0 0 1 2 2 2
  spline S107 degree 2 poles (28.1633, 40.9376) (28.1633, 41.1988) (27.9172, 41.5358) (27.671, 41.6343) knots 0 0 0 1 2 2 2
  spline S108 degree 2 poles (27.671, 41.6343) (27.4325, 41.729) (26.7055, 41.7971) (26.2473, 41.7971) knots 0 0 0 1 2 2 2
  spline S109 degree 2 poles (26.2473, 41.7971) (25.755, 41.7971) (25.0962, 41.7365) (24.8387, 41.6381) knots 0 0 0 1 2 2 2
  spline S110 degree 2 poles (24.8387, 41.6381) (24.5964, 41.5472) (24.3351, 41.2102) (24.3351, 40.9376) knots 0 0 0 1 2 2 2
  spline S111 degree 2 poles (24.3351, 40.9376) (24.3351, 40.6801) (24.5812, 40.3431) (24.8273, 40.2484) knots 0 0 0 1 2 2 2
  line L125 (16.2215, 89.5737) -> (20.8941, 87.9985)
  line L126 (20.8941, 87.9985) -> (20.8941, 87.2336)
  line L127 (20.8941, 87.2336) -> (16.2215, 85.6584)
  line L128 (16.2215, 85.6584) -> (16.2215, 86.3135)
  line L129 (16.2215, 86.3135) -> (17.5279, 86.7376)
  line L130 (17.5279, 86.7376) -> (17.5279, 88.5211)
  line L131 (17.5279, 88.5211) -> (16.2215, 88.9452)
  line L132 (16.2215, 88.9452) -> (16.2215, 89.5737)
  line L133 (18.058, 86.908) -> (20.2579, 87.6312)
  line L134 (20.2579, 87.6312) -> (18.058, 88.3507)
  line L135 (18.058, 88.3507) -> (18.058, 86.908)
  line L136 (19.0955, 83.4017) -> (19.0955, 83.432)
  spline S112 degree 2 poles (19.0955, 83.432) (19.1144, 83.5001) (19.122, 83.6478) (19.122, 83.75) knots 0 0 0 1 2 2 2
  spline S113 degree 2 poles (19.122, 83.75) (19.122, 83.9886) (18.9137, 84.4581) (18.7093, 84.6702) knots 0 0 0 1 2 2 2
  line L137 (18.7093, 84.6702) -> (16.2215, 84.6702)
  line L138 (16.2215, 84.6702) -> (16.2215, 85.2609)
  line L139 (16.2215, 85.2609) -> (19.7278, 85.2609)
  line L140 (19.7278, 85.2609) -> (19.7278, 84.6702)
  line L141 (19.7278, 84.6702) -> (19.2053, 84.6702)
  spline S114 degree 2 poles (19.2053, 84.6702) (19.4931, 84.3483) (19.7278, 83.8674) (19.7278, 83.6402) knots 0 0 0 1 2 2 2
  spline S115 degree 2 poles (19.7278, 83.6402) (19.7278, 83.5493) (19.7203, 83.4585) (19.7089, 83.4017) knots 0 0 0 1 2 2 2
  line L142 (19.7089, 83.4017) -> (19.0955, 83.4017)
  line L143 (16.2215, 80.2475) -> (16.2215, 80.8382)
  line L144 (16.2215, 80.8382) -> (16.5774, 80.8382)
  spline S116 degree 2 poles (16.5774, 80.8382) (16.4638, 80.9745) (16.3124, 81.1752) (16.248, 81.3115) knots 0 0 0 1 2 2 2
  spline S117 degree 2 poles (16.248, 81.3115) (16.1874, 81.4365) (16.123, 81.7053) (16.123, 81.8833) knots 0 0 0 1 2 2 2
  spline S118 degree 2 poles (16.123, 81.8833) (16.123, 82.171) (16.3616, 82.6557) (16.5926, 82.8261) knots 0 0 0 1 2 2 2
  spline S119 degree 2 poles (16.5926, 82.8261) (16.8236, 82.9965) (17.5051, 83.1858) (17.9482, 83.1858) knots 0 0 0 1 2 2 2
  spline S120 degree 2 poles (17.9482, 83.1858) (18.4101, 83.1858) (19.0841, 82.9473) (19.3378, 82.739) knots 0 0 0 1 2 2 2
  spline S121 degree 2 poles (19.3378, 82.739) (19.565, 82.5459) (19.8263, 82.0044) (19.8263, 81.7053) knots 0 0 0 1 2 2 2
  spline S122 degree 2 poles (19.8263, 81.7053) (19.8263, 81.444) (19.7089, 81.054) (19.5877, 80.8382) knots 0 0 0 1 2 2 2
  line L145 (19.5877, 80.8382) -> (21.1023, 80.8382)
  line L146 (21.1023, 80.8382) -> (21.1023, 80.2475)
  line L147 (21.1023, 80.2475) -> (16.2215, 80.2475)
  line L148 (17.0735, 80.8382) -> (19.0993, 80.8382)
  spline S123 degree 2 poles (19.0993, 80.8382) (19.2053, 81.0578) (19.2848, 81.4062) (19.2848, 81.6069) knots 0 0 0 1 2 2 2
  spline S124 degree 2 poles (19.2848, 81.6069) (19.2848, 82.0612) (18.6032, 82.5762) (17.9595, 82.5762) knots 0 0 0 1 2 2 2
  spline S125 degree 2 poles (17.9595, 82.5762) (17.3385, 82.5762) (16.6835, 82.1824) (16.6835, 81.747) knots 0 0 0 1 2 2 2
  spline S126 degree 2 poles (16.6835, 81.747) (16.6835, 81.516) (16.8955, 81.0464) (17.0735, 80.8382) knots 0 0 0 1 2 2 2
  line L149 (16.2215, 76.6654) -> (16.2215, 77.2561)
  line L150 (16.2215, 77.2561) -> (16.6077, 77.2561)
  spline S127 degree 2 poles (16.6077, 77.2561) (16.3692, 77.5288) (16.123, 78.0172) (16.123, 78.3201) knots 0 0 0 1 2 2 2
  spline S128 degree 2 poles (16.123, 78.3201) (16.123, 78.5473) (16.2745, 78.9525) (16.4373, 79.1002) knots 0 0 0 1 2 2 2
  spline S129 degree 2 poles (16.4373, 79.1002) (16.6002, 79.2516) (17.0962, 79.4182) (17.4521, 79.4182) knots 0 0 0 1 2 2 2
  line L151 (17.4521, 79.4182) -> (19.7278, 79.4182)
  line L152 (19.7278, 79.4182) -> (19.7278, 78.8275)
  line L153 (19.7278, 78.8275) -> (17.7285, 78.8275)
  spline S130 degree 2 poles (17.7285, 78.8275) (17.4483, 78.8275) (17.081, 78.7859) (16.9447, 78.7139) knots 0 0 0 1 2 2 2
  spline S131 degree 2 poles (16.9447, 78.7139) (16.8084, 78.642) (16.6835, 78.3959) (16.6835, 78.1649) knots 0 0 0 1 2 2 2
  spline S132 degree 2 poles (16.6835, 78.1649) (16.6835, 77.9491) (16.9296, 77.4606) (17.1075, 77.2561) knots 0 0 0 1 2 2 2
  line L154 (17.1075, 77.2561) -> (19.7278, 77.2561)
  line L155 (19.7278, 77.2561) -> (19.7278, 76.6654)
  line L156 (19.7278, 76.6654) -> (16.2215, 76.6654)
  line L157 (16.2215, 75.2076) -> (16.2215, 75.7983)
  line L158 (16.2215, 75.7983) -> (19.7278, 75.7983)
  line L159 (19.7278, 75.7983) -> (19.7278, 75.2076)
  line L160 (19.7278, 75.2076) -> (16.2215, 75.2076)
  line L161 (20.311, 75.166) -> (20.311, 75.8362)
  line L162 (20.311, 75.8362) -> (20.9244, 75.8362)
  line L163 (20.9244, 75.8362) -> (20.9244, 75.166)
  line L164 (20.9244, 75.166) -> (20.311, 75.166)
  line L165 (16.2215, 71.5877) -> (16.2215, 72.1784)
  line L166 (16.2215, 72.1784) -> (18.2208, 72.1784)
  spline S133 degree 2 poles (18.2208, 72.1784) (18.4631, 72.1784) (18.8796, 72.2238) (19.0046, 72.292) knots 0 0 0 1 2 2 2
  spline S134 degree 2 poles (19.0046, 72.292) (19.1371, 72.3639) (19.2659, 72.6214) (19.2659, 72.841) knots 0 0 0 1 2 2 2
  spline S135 degree 2 poles (19.2659, 72.841) (19.2659, 73.0606) (19.0311, 73.5264) (18.8418, 73.7498) knots 0 0 0 1 2 2 2
  line L167 (18.8418, 73.7498) -> (16.2215, 73.7498)
  line L168 (16.2215, 73.7498) -> (16.2215, 74.3405)
  line L169 (16.2215, 74.3405) -> (19.7278, 74.3405)
  line L170 (19.7278, 74.3405) -> (19.7278, 73.7498)
  line L171 (19.7278, 73.7498) -> (19.3378, 73.7498)
  spline S136 degree 2 poles (19.3378, 73.7498) (19.5764, 73.4847) (19.8263, 72.9736) (19.8263, 72.6858) knots 0 0 0 1 2 2 2
  spline S137 degree 2 poles (19.8263, 72.6858) (19.8263, 72.1708) (19.1447, 71.5877) (18.4972, 71.5877) knots 0 0 0 1 2 2 2
  line L172 (18.4972, 71.5877) -> (16.2215, 71.5877)
  spline S138 degree 2 poles (17.9747, 67.8769) (17.0886, 67.8769) (16.123, 68.7288) (16.123, 69.4407) knots 0 0 0 1 2 2 2
  spline S139 degree 2 poles (16.123, 69.4407) (16.123, 70.1715) (17.1189, 71.0083) (17.9747, 71.0083) knots 0 0 0 1 2 2 2
  spline S140 degree 2 poles (17.9747, 71.0083) (18.8531, 71.0083) (19.8263, 70.145) (19.8263, 69.4407) knots 0 0 0 1 2 2 2
  spline S141 degree 2 poles (19.8263, 69.4407) (19.8263, 68.7288) (18.8569, 67.8769) (17.9747, 67.8769) knots 0 0 0 1 2 2 2
  spline S142 degree 2 poles (17.9747, 68.4865) (18.6562, 68.4865) (19.3189, 68.9825) (19.3189, 69.4407) knots 0 0 0 1 2 2 2
  spline S143 degree 2 poles (19.3189, 69.4407) (19.3189, 69.8989) (18.6562, 70.3987) (17.9747, 70.3987) knots 0 0 0 1 2 2 2
  spline S144 degree 2 poles (17.9747, 70.3987) (17.312, 70.3987) (16.6304, 69.8989) (16.6304, 69.4407) knots 0 0 0 1 2 2 2
  spline S145 degree 2 poles (16.6304, 69.4407) (16.6304, 68.9863) (17.3007, 68.4865) (17.9747, 68.4865) knots 0 0 0 1 2 2 2
  line L173 (16.2215, 65.2187) -> (20.8941, 65.2187)
  line L174 (20.8941, 65.2187) -> (20.8941, 62.2955)
  line L175 (20.8941, 62.2955) -> (20.3412, 62.2955)
  line L176 (20.3412, 62.2955) -> (20.3412, 64.5977)
  line L177 (20.3412, 64.5977) -> (19.0614, 64.5977)
  line L178 (19.0614, 64.5977) -> (19.0614, 62.4508)
  line L179 (19.0614, 62.4508) -> (18.5086, 62.4508)
  line L180 (18.5086, 62.4508) -> (18.5086, 64.5977)
  line L181 (18.5086, 64.5977) -> (16.7743, 64.5977)
  line L182 (16.7743, 64.5977) -> (16.7743, 62.2955)
  line L183 (16.7743, 62.2955) -> (16.2215, 62.2955)
  line L184 (16.2215, 62.2955) -> (16.2215, 65.2187)
  line L185 (16.2215, 58.9634) -> (16.2215, 59.5541)
  line L186 (16.2215, 59.5541) -> (16.5774, 59.5541)
  spline S146 degree 2 poles (16.5774, 59.5541) (16.4638, 59.6904) (16.3124, 59.8911) (16.248, 60.0274) knots 0 0 0 1 2 2 2
  spline S147 degree 2 poles (16.248, 60.0274) (16.1874, 60.1523) (16.123, 60.4212) (16.123, 60.5992) knots 0 0 0 1 2 2 2
  spline S148 degree 2 poles (16.123, 60.5992) (16.123, 60.8869) (16.3616, 61.3716) (16.5926, 61.542) knots 0 0 0 1 2 2 2
  spline S149 degree 2 poles (16.5926, 61.542) (16.8236, 61.7124) (17.5051, 61.9017) (17.9482, 61.9017) knots 0 0 0 1 2 2 2
  spline S150 degree 2 poles (17.9482, 61.9017) (18.4101, 61.9017) (19.0841, 61.6632) (19.3378, 61.4549) knots 0 0 0 1 2 2 2
  spline S151 degree 2 poles (19.3378, 61.4549) (19.565, 61.2618) (19.8263, 60.7203) (19.8263, 60.4212) knots 0 0 0 1 2 2 2
  spline S152 degree 2 poles (19.8263, 60.4212) (19.8263, 60.1599) (19.7089, 59.7699) (19.5877, 59.5541) knots 0 0 0 1 2 2 2
  line L187 (19.5877, 59.5541) -> (21.1023, 59.5541)
  line L188 (21.1023, 59.5541) -> (21.1023, 58.9634)
  line L189 (21.1023, 58.9634) -> (16.2215, 58.9634)
  line L190 (17.0735, 59.5541) -> (19.0993, 59.5541)
  spline S153 degree 2 poles (19.0993, 59.5541) (19.2053, 59.7737) (19.2848, 60.1221) (19.2848, 60.3227) knots 0 0 0 1 2 2 2
  spline S154 degree 2 poles (19.2848, 60.3227) (19.2848, 60.7771) (18.6032, 61.2921) (17.9595, 61.2921) knots 0 0 0 1 2 2 2
  spline S155 degree 2 poles (17.9595, 61.2921) (17.3385, 61.2921) (16.6835, 60.8983) (16.6835, 60.4628) knots 0 0 0 1 2 2 2
  spline S156 degree 2 poles (16.6835, 60.4628) (16.6835, 60.2319) (16.8955, 59.7623) (17.0735, 59.5541) knots 0 0 0 1 2 2 2
  line L191 (16.2215, 57.5056) -> (16.2215, 58.0963)
  line L192 (16.2215, 58.0963) -> (19.7278, 58.0963)
  line L193 (19.7278, 58.0963) -> (19.7278, 57.5056)
  line L194 (19.7278, 57.5056) -> (16.2215, 57.5056)
  line L195 (20.311, 57.4639) -> (20.311, 58.1341)
  line L196 (20.311, 58.1341) -> (20.9244, 58.1341)
  line L197 (20.9244, 58.1341) -> (20.9244, 57.4639)
  line L198 (20.9244, 57.4639) -> (20.311, 57.4639)
  spline S157 degree 2 poles (16.1533, 55.5782) (16.1533, 56.0591) (16.7024, 56.6006) (17.2969, 56.6006) knots 0 0 0 1 2 2 2
  line L199 (17.2969, 56.6006) -> (19.2394, 56.6006)
  line L200 (19.2394, 56.6006) -> (19.2394, 56.9982)
  line L201 (19.2394, 56.9982) -> (19.7278, 56.9982)
  line L202 (19.7278, 56.9982) -> (19.7278, 56.6006)
  line L203 (19.7278, 56.6006) -> (20.735, 56.6006)
  line L204 (20.735, 56.6006) -> (20.735, 56.0099)
  line L205 (20.735, 56.0099) -> (19.7278, 56.0099)
  line L206 (19.7278, 56.0099) -> (19.7278, 54.9231)
  line L207 (19.7278, 54.9231) -> (19.2394, 54.9231)
  line L208 (19.2394, 54.9231) -> (19.2394, 56.0099)
  line L209 (19.2394, 56.0099) -> (17.5695, 56.0099)
  spline S158 degree 2 poles (17.5695, 56.0099) (17.3044, 56.0099) (17.0129, 55.9909) (16.8879, 55.9266) knots 0 0 0 1 2 2 2
  spline S159 degree 2 poles (16.8879, 55.9266) (16.7781, 55.8736) (16.6683, 55.635) (16.6683, 55.4305) knots 0 0 0 1 2 2 2
  spline S160 degree 2 poles (16.6683, 55.4305) (16.6683, 55.2866) (16.7554, 55.0178) (16.7819, 54.9572) knots 0 0 0 1 2 2 2
  line L210 (16.7819, 54.9572) -> (16.7819, 54.9231)
  line L211 (16.7819, 54.9231) -> (16.2518, 54.9231)
  spline S161 degree 2 poles (16.2518, 54.9231) (16.2064, 55.0897) (16.1533, 55.4305) (16.1533, 55.5782) knots 0 0 0 1 2 2 2
  line L212 (16.2215, 53.8856) -> (16.2215, 54.4763)
  line L213 (16.2215, 54.4763) -> (19.7278, 54.4763)
  line L214 (19.7278, 54.4763) -> (19.7278, 53.8856)
  line L215 (19.7278, 53.8856) -> (16.2215, 53.8856)
  line L216 (20.311, 53.844) -> (20.311, 54.5142)
  line L217 (20.311, 54.5142) -> (20.9244, 54.5142)
  line L218 (20.9244, 54.5142) -> (20.9244, 53.844)
  line L219 (20.9244, 53.844) -> (20.311, 53.844)
  spline S162 degree 2 poles (17.9747, 50.137) (17.0886, 50.137) (16.123, 50.9889) (16.123, 51.7008) knots 0 0 0 1 2 2 2
  spline S163 degree 2 poles (16.123, 51.7008) (16.123, 52.4316) (17.1189, 53.2684) (17.9747, 53.2684) knots 0 0 0 1 2 2 2
  spline S164 degree 2 poles (17.9747, 53.2684) (18.8531, 53.2684) (19.8263, 52.4051) (19.8263, 51.7008) knots 0 0 0 1 2 2 2
  spline S165 degree 2 poles (19.8263, 51.7008) (19.8263, 50.9889) (18.8569, 50.137) (17.9747, 50.137) knots 0 0 0 1 2 2 2
  spline S166 degree 2 poles (17.9747, 50.7466) (18.6562, 50.7466) (19.3189, 51.2426) (19.3189, 51.7008) knots 0 0 0 1 2 2 2
  spline S167 degree 2 poles (19.3189, 51.7008) (19.3189, 52.159) (18.6562, 52.6588) (17.9747, 52.6588) knots 0 0 0 1 2 2 2
  spline S168 degree 2 poles (17.9747, 52.6588) (17.312, 52.6588) (16.6304, 52.159) (16.6304, 51.7008) knots 0 0 0 1 2 2 2
  spline S169 degree 2 poles (16.6304, 51.7008) (16.6304, 51.2464) (17.3007, 50.7466) (17.9747, 50.7466) knots 0 0 0 1 2 2 2
  line L220 (16.2215, 46.7783) -> (16.2215, 47.369)
  line L221 (16.2215, 47.369) -> (18.2208, 47.369)
  spline S170 degree 2 poles (18.2208, 47.369) (18.4631, 47.369) (18.8796, 47.4144) (19.0046, 47.4826) knots 0 0 0 1 2 2 2
  spline S171 degree 2 poles (19.0046, 47.4826) (19.1371, 47.5545) (19.2659, 47.812) (19.2659, 48.0316) knots 0 0 0 1 2 2 2
  spline S172 degree 2 poles (19.2659, 48.0316) (19.2659, 48.2513) (19.0311, 48.717) (18.8418, 48.9404) knots 0 0 0 1 2 2 2
  line L222 (18.8418, 48.9404) -> (16.2215, 48.9404)
  line L223 (16.2215, 48.9404) -> (16.2215, 49.5311)
  line L224 (16.2215, 49.5311) -> (19.7278, 49.5311)
  line L225 (19.7278, 49.5311) -> (19.7278, 48.9404)
  line L226 (19.7278, 48.9404) -> (19.3378, 48.9404)
  spline S173 degree 2 poles (19.3378, 48.9404) (19.5764, 48.6754) (19.8263, 48.1642) (19.8263, 47.8764) knots 0 0 0 1 2 2 2
  spline S174 degree 2 poles (19.8263, 47.8764) (19.8263, 47.3614) (19.1447, 46.7783) (18.4972, 46.7783) knots 0 0 0 1 2 2 2
  line L227 (18.4972, 46.7783) -> (16.2215, 46.7783)
  spline S175 degree 2 poles (8.4487, 102.713) (8.4487, 103.5536) (9.3915, 104.4775) (10.2624, 104.4775) knots 0 0 0 1 2 2 2
  spline S176 degree 2 poles (10.2624, 104.4775) (11.1182, 104.4775) (12.133, 103.5801) (12.133, 102.8569) knots 0 0 0 1 2 2 2
  spline S177 degree 2 poles (12.133, 102.8569) (12.133, 102.5312) (11.9437, 102.0276) (11.743, 101.8421) knots 0 0 0 1 2 2 2
  spline S178 degree 2 poles (11.743, 101.8421) (11.5423, 101.6528) (10.963, 101.4521) (10.5426, 101.4521) knots 0 0 0 1 2 2 2
  line L228 (10.5426, 101.4521) -> (10.2208, 101.4521)
  line L229 (10.2208, 101.4521) -> (10.2208, 103.8792)
  spline S179 degree 2 poles (10.2208, 103.8792) (9.6112, 103.8792) (8.9637, 103.2658) (8.9637, 102.7206) knots 0 0 0 1 2 2 2
  spline S180 degree 2 poles (8.9637, 102.7206) (8.9637, 102.5275) (9.0508, 102.1526) (9.1189, 102.0011) knots 0 0 0 1 2 2 2
  spline S181 degree 2 poles (9.1189, 102.0011) (9.1946, 101.8421) (9.3272, 101.6225) (9.3878, 101.5505) knots 0 0 0 1 2 2 2
  line L230 (9.3878, 101.5505) -> (9.3878, 101.5165)
  line L231 (9.3878, 101.5165) -> (8.744, 101.5165)
  spline S182 degree 2 poles (8.744, 101.5165) (8.7024, 101.6187) (8.5812, 101.9292) (8.5471, 102.0504) knots 0 0 0 1 2 2 2
  spline S183 degree 2 poles (8.5471, 102.0504) (8.4979, 102.2207) (8.4487, 102.5009) (8.4487, 102.713) knots 0 0 0 1 2 2 2
  spline S184 degree 2 poles (10.6714, 102.0276) (10.9099, 102.0352) (11.2583, 102.1337) (11.3757, 102.2283) knots 0 0 0 1 2 2 2
  spline S185 degree 2 poles (11.3757, 102.2283) (11.5082, 102.3306) (11.6483, 102.6524) (11.6483, 102.891) knots 0 0 0 1 2 2 2
  spline S186 degree 2 poles (11.6483, 102.891) (11.6483, 103.1257) (11.5082, 103.4552) (11.3719, 103.5915) knots 0 0 0 1 2 2 2
  spline S187 degree 2 poles (11.3719, 103.5915) (11.2318, 103.724) (10.8948, 103.8603) (10.6714, 103.8792) knots 0 0 0 1 2 2 2
  line L232 (10.6714, 103.8792) -> (10.6714, 102.0276)
  line L233 (8.5282, 98.101) -> (8.5282, 98.6917)
  line L234 (8.5282, 98.6917) -> (10.5275, 98.6917)
  spline S188 degree 2 poles (10.5275, 98.6917) (10.7698, 98.6917) (11.1864, 98.7371) (11.3113, 98.8053) knots 0 0 0 1 2 2 2
  spline S189 degree 2 poles (11.3113, 98.8053) (11.4438, 98.8772) (11.5726, 99.1347) (11.5726, 99.3543) knots 0 0 0 1 2 2 2
  spline S190 degree 2 poles (11.5726, 99.3543) (11.5726, 99.574) (11.3378, 100.0397) (11.1485, 100.2631) knots 0 0 0 1 2 2 2
  line L235 (11.1485, 100.2631) -> (8.5282, 100.2631)
  line L236 (8.5282, 100.2631) -> (8.5282, 100.8538)
  line L237 (8.5282, 100.8538) -> (12.0345, 100.8538)
  line L238 (12.0345, 100.8538) -> (12.0345, 100.2631)
  line L239 (12.0345, 100.2631) -> (11.6445, 100.2631)